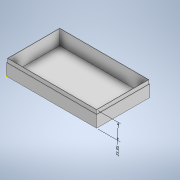
# Autodesk Inventor part: tapa
Saved by Autodesk Inventor 2022 (Build 260153000, 153)
## iProperties
Created: 2021-05-28
Part Number: tapa
Material: Generic
Document SubType Name: Modeling
Designer: Pau
Density: 1 g/cm^3
Appearance: Default
Author: Pau
Autodesk Inventor part; units mm, degrees
ref_plane "YZ Plane" through (0, 0, 0) normal (1, 0, 0) x (0, 1, 0)
ref_plane "XZ Plane" through (0, 0, 0) normal (0, 1, 0) x (-1, 0, 0)
ref_plane "XY Plane" through (0, 0, 0) normal (0, 0, 1) x (1, 0, 0)
sketch "Sketch1" plane through (0, 0, 0) normal (0, 1, 0) x (-1, 0, 0)
  point P0 (0, 0)
sketch "Sketch2" plane through (0, 0, 0) normal (0, 1, 0) x (-1, 0, 0)
  line L0 (0, 0) -> (-122, 0)
  line L1 (-122, 0) -> (-122, -72)
  line L2 (-122, -72) -> (0, -72)
  line L3 (0, -72) -> (0, 0)
  dimension "d0" = 122
  dimension "d1" = 72
  constraints: 8 end point, 2 parallel, 1 horizontal, 1 perpendicular
  measures "d0" distance of L2.end L1.end
  measures "d1" distance of L1.end L0.end
extrude "Extrusion1" add sketch "Sketch2" along normal blind 1
sketch "Sketch3" plane through (0, 1, 0) normal (0, 1, 0) x (1, 0, 0)
  line L0 (122, 72) -> (0, 72) projected
  line L1 (0, 72) -> (1, 72)
  line L2 (1, 72) -> (1, 71)
  line L3 (1, 71) -> (0, 71)
  line L4 (0, 71) -> (0, 72)
  line L5 (122, 0) -> (122, 72) projected
  line L6 (122, 0) -> (121, 0)
  line L7 (121, 0) -> (121, 1)
  line L8 (121, 1) -> (122, 1)
  line L9 (122, 1) -> (122, 0)
  line L10 (1, 71) -> (121, 71)
  line L11 (121, 71) -> (121, 1)
  line L12 (121, 1) -> (1, 1)
  line L13 (1, 1) -> (1, 71)
  line L14 (0, 71) -> (122, 71)
  line L15 (122, 71) -> (122, 0)
  line L16 (122, 0) -> (0, 0)
  line L17 (0, 0) -> (0, 71)
  dimension "d4" = 1
  dimension "d5" = 1
  dimension "d6" = 1
  dimension "d7" = 1
  constraints: 32 end point, 8 parallel, 4 horizontal, 4 perpendicular
  measures "d4" distance of L2.end L3.end
  measures "d5" distance of L1.end L2.end
  measures "d6" distance of L7.end L8.end
  measures "d7" distance of L6.end L7.end
extrude "Extrusion2" add sketch "Sketch3" along normal blind 15 contours L5 L14 L10 L2 L0 | L2 L3 L4 L0 | L5 L8 L11 L14 | L13 L12 L7 L16 L17 L3 | L5 L6 L7 L8
sketch "Sketch5" plane through (0, 16, 0) normal (0, 1, 0) x (1, 0, 0)
  line L0 (0, 0) -> (122, 0) projected
  line L1 (0, 0) -> (0.5, 0)
  line L2 (0.5, 0) -> (0.5, 0.5)
  line L3 (0.5, 0.5) -> (0, 0.5)
  line L4 (0, 0.5) -> (0, 0)
  line L5 (122, 72) -> (121.5, 72)
  line L6 (121.5, 72) -> (121.5, 71.5)
  line L7 (121.5, 71.5) -> (122, 71.5)
  line L8 (122, 71.5) -> (122, 72)
  line L9 (121.5, 71.5) -> (0.5, 71.5)
  line L10 (0.5, 71.5) -> (0.5, 0.5)
  line L11 (0.5, 0.5) -> (121.5, 0.5)
  line L12 (121.5, 0.5) -> (121.5, 71.5)
  line L13 (121, 71) -> (121, 1) projected
  line L14 (1, 1) -> (1, 71) projected
  line L15 (121, 1) -> (1, 1)
  line L16 (1, 1) -> (1, 71)
  line L17 (1, 71) -> (121, 71)
  line L18 (121, 71) -> (121, 1)
  point P0 (121, 71)
  dimension "d10" = 0.5
  dimension "d11" = 0.5
  dimension "d12" = 0.5
  dimension "d13" = 0.5
  constraints: 32 end point, 8 parallel, 4 horizontal, 4 perpendicular
  measures "d10" distance of L3.end L2.end
  measures "d11" distance of L2.end L1.end
  measures "d12" distance of L7.end L6.end
  measures "d13" distance of L6.end L5.end
extrude "Extrusion3" add sketch "Sketch5" along normal blind 5 contours L10 L9 L12 L11
body "Solid1"
